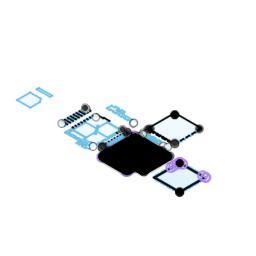
pccases (Autodesk Fusion 360 design; units mm, degrees)
Autodesk Fusion 360 part; units mm, degrees
note: some values were not read from the file. Chosen so that the rebuilt part matches the saved one: which pieces of a blend or face edit are solid.
(part 1 of 5)
sketch "Skizze1" plane through (0, 0, 0) normal (0, 0, 1) x (1, 0, 0)
  line L0 (240, 0) -> (240, 8)
  line L1 (240, 8) -> (10, 8)
  line L2 (10, 8) -> (10, 0)
  line L3 (10.0001, -328) -> (10.0001, -331)
  line L4 (0.0001, -331) -> (0.0001, -328)
  line L5 (250, -328) -> (250, -331)
  line L6 (240, -331) -> (240, -328)
  circle A0 centre (7.5, -7.5) radius 1.5
  circle A1 centre (7.5, -242.5) radius 1.5
  circle A2 centre (242.5, -242.5) radius 1.5
  line L7 (0, 0) -> (10, 0)
  line L8 (0, 0) -> (10, 0)
  line L9 (240, 0) -> (250, 0)
  line L10 (240, -328) -> (10.0001, -328)
  line L11 (10.5, -10.5) -> (239.5, -10.5)
  line L12 (239.5, -10.5) -> (239.5, -239.5)
  line L13 (239.5, -239.5) -> (10.5, -239.5)
  line L14 (10.5, -239.5) -> (10.5, -10.5)
  line L15 (0, -250) -> (-8, -250)
  line L16 (250, -258) -> (250, -250)
  circle A3 centre (-15.5, -7.5) radius 1.5
  circle A4 centre (7.5, -265.5) radius 1.5
  circle A5 centre (242.5, -265.5) radius 1.5
  circle A6 centre (7.5, -320.5) radius 1.5
  circle A7 centre (242.5, -320.5) radius 1.5
  circle A8 centre (-15.5, -242.5) radius 1.5
  circle A9 centre (-70.5, -242.5) radius 1.5
  line L17 (-15, -250) -> (-15, -258)
  line L18 (-15, -258) -> (-22, -258)
  line L19 (-22, -258) -> (-22, -250)
  line L20 (0.0075, -258) -> (-7.9925, -258)
  line L21 (-7.9925, -258) -> (-7.9925, -265)
  line L22 (-7.9925, -265) -> (0, -265)
  line L23 (250, -258) -> (258, -258)
  line L24 (258, -268) -> (250, -268)
  line L25 (250, -250) -> (250, -258)
  line L26 (-15, -250) -> (-8, -250)
  line L27 (-8, -272) -> (-8, -279)
  line L28 (-8, -279) -> (0, -279)
  line L29 (0, -272) -> (-8, -272)
  line L30 (-8, -286) -> (-8, -293)
  line L31 (-8, -293) -> (0, -293)
  line L32 (0, -286) -> (-8, -286)
  line L33 (-8, -300) -> (-8, -307)
  line L34 (-8, -307) -> (0, -307)
  line L35 (0, -300) -> (-8, -300)
  line L36 (-8, -314) -> (-8, -321)
  line L37 (-8, -321) -> (0.0001, -321)
  line L38 (0, -314) -> (-8, -314)
  line L39 (-29, -258) -> (-36, -258)
  line L40 (-36, -258) -> (-36, -250)
  line L41 (-29, -250) -> (-29, -258)
  line L42 (-43, -258) -> (-50, -258)
  line L43 (-50, -258) -> (-50, -250)
  line L44 (-43, -250) -> (-43, -258)
  line L45 (-57, -258) -> (-64, -258)
  line L46 (-64, -258) -> (-64, -250)
  line L47 (-57, -250) -> (-57, -258)
  line L48 (-71, -258) -> (-78, -258)
  line L49 (-78, -258) -> (-78, -250)
  line L50 (-71, -250) -> (-71, -258)
  line L51 (0, -272) -> (0, -265)
  line L52 (0, -286) -> (0, -279)
  line L53 (0, -314) -> (0, -307)
  line L54 (0, -300) -> (0, -293)
  line L55 (250, -318) -> (250, -328)
  line L56 (250, -250) -> (250, -258)
  line L57 (0, 0) -> (-8, 0)
  line L58 (-8, -250) -> (0, -250)
  line L59 (-71, -250) -> (-64, -250)
  line L60 (-57, -250) -> (-50, -250)
  line L61 (-43, -250) -> (-36, -250)
  line L62 (-29, -250) -> (-22, -250)
  line L63 (0, 0) -> (-8, 0)
  line L64 (-78, 8) -> (-8, 8)
  line L65 (250, -250) -> (250, -258)
  line L66 (-18.5, -10.5) -> (-67.5, -10.5)
  line L67 (-67.5, -10.5) -> (-67.5, -239.5)
  line L68 (-67.5, -239.5) -> (-18.5, -239.5)
  line L69 (-18.5, -239.5) -> (-18.5, -10.5)
  circle A10 centre (-70.5, -7.5) radius 1.5
  line L70 (-113.0202, -27.7778) -> (-121, -27.7778)
  line L71 (-113.0173, -55.5556) -> (-121, -55.5556)
  line L72 (-113.0145, -83.3367) -> (-121, -83.3367)
  line L73 (-113.0116, -111.1141) -> (-121, -111.1141)
  line L74 (-113.0087, -138.888) -> (-121, -138.888)
  line L75 (-113.0058, -166.6654) -> (-121, -166.6654)
  line L76 (-113.0029, -194.4429) -> (-121, -194.4429)
  line L77 (-113, -222.2215) -> (-121, -222.2224)
  line L78 (-370.8329, -27.7778) -> (-378.9302, -27.7778)
  line L79 (-370.8329, -55.5556) -> (-378.9302, -55.5556)
  line L80 (-370.8329, -83.3333) -> (-378.9302, -83.3333)
  line L81 (-370.8329, -138.8889) -> (-378.9302, -138.8889)
  line L82 (-370.8329, -166.6667) -> (-378.9302, -166.6667)
  line L83 (-370.8329, -194.4444) -> (-378.9302, -194.4444)
  line L84 (-370.8329, -222.2222) -> (-378.9302, -222.2222)
  line L85 (0, -250) -> (27.7778, -250)
  line L86 (55.5556, -250) -> (83.3333, -250)
  line L87 (111.1111, -250) -> (138.8889, -250)
  line L88 (166.6667, -250) -> (194.4444, -250)
  line L89 (222.2222, -250) -> (250, -250)
  line L90 (-121, -255.9081) -> (-121, -222.2224)
  line L91 (-121, -255.9081) -> (-121, -222.2224)
  line L92 (-121, -194.4429) -> (-121, -166.6654)
  line L93 (-121, -194.4429) -> (-121, -166.6654)
  line L94 (-121, -138.888) -> (-121, -111.1141)
  line L95 (-121, -83.3367) -> (-121, -55.5556)
  line L96 (-121, -138.888) -> (-121, -111.1141)
  line L97 (-121, -83.3367) -> (-121, -55.5556)
  line L98 (-121, -27.7778) -> (-121, 0)
  line L99 (-370.8329, 0) -> (-370.8329, -27.7778)
  line L100 (-370.8329, -55.5556) -> (-370.8329, -83.3333)
  line L101 (-370.8329, -111.1111) -> (-370.8329, -138.8889)
  line L102 (-370.8329, -166.6667) -> (-370.8329, -194.4444)
  line L103 (-370.8329, -222.2222) -> (-370.8329, -263.9081)
  line L104 (10.5, -268.5) -> (239.5, -268.5)
  line L105 (239.5, -268.5) -> (239.5, -317.5)
  line L106 (239.5, -317.5) -> (10.5, -317.5)
  line L107 (10.5, -317.5) -> (10.5, -268.5)
  line L108 (0.0001, -321) -> (0.0001, -328)
  line L109 (0, -27.7778) -> (-8, -27.7778)
  line L110 (0, -55.5556) -> (-8, -55.5556)
  line L111 (0, -83.3333) -> (-8, -83.3333)
  line L112 (0, -111.1111) -> (-8, -111.1111)
  line L113 (0, -138.8889) -> (-8, -138.8889)
  line L114 (0, -166.6667) -> (-8, -166.6667)
  line L115 (0, -194.4444) -> (-8, -194.4444)
  line L116 (0, -222.2222) -> (-8, -222.2222)
  line L117 (0, -250) -> (-8, -250)
  line L118 (-8, -27.7778) -> (-8, -55.5556)
  line L119 (-8, -83.3333) -> (-8, -111.1111)
  line L120 (-8, -138.8889) -> (-8, -166.6667)
  line L121 (-8, -194.4444) -> (-8, -222.2222)
  line L122 (0, -222.2222) -> (0.0075, -258)
  line L123 (0, -111.1111) -> (0, -138.8889)
  line L124 (0, -166.6667) -> (0, -194.4444)
  line L125 (0, 0) -> (0, -27.7778)
  line L126 (0, -55.5556) -> (0, -83.3333)
  line L127 (-78, -27.7778) -> (-86, -27.7778)
  line L128 (-78, -55.5556) -> (-86, -55.5556)
  line L129 (-78, -83.3333) -> (-86, -83.3333)
  line L130 (-78, -111.1111) -> (-86, -111.1111)
  line L131 (-78, -138.8889) -> (-86, -138.8889)
  line L132 (-78, -166.6667) -> (-86, -166.6667)
  line L133 (-78, -194.4444) -> (-86, -194.4444)
  line L134 (-78, -222.2222) -> (-86, -222.2222)
  line L135 (-355.7398, -242.9081) -> (-228.7398, -242.9081)
  line L136 (-228.7398, -242.9081) -> (-228.7398, -263.9081)
  line L137 (-355.7398, -263.9081) -> (-355.7398, -242.9081)
  line L138 (-253.6584, -13) -> (-253.6584, 8)
  line L139 (-126.6584, -0.0224) -> (-126.6584, -13)
  line L140 (-126.6584, -13) -> (-253.6584, -13)
  line L141 (-355.7398, -116.9081) -> (-253.7398, -116.9081)
  line L142 (-228.7398, -152.9081) -> (-228.7398, -242.9081)
  line L143 (-228.7398, -242.9081) -> (-355.7398, -242.9081)
  line L144 (-355.7398, -242.9081) -> (-355.7398, -116.9081)
  line L145 (-253.7398, -116.9081) -> (-228.7398, -152.9081)
  line L146 (-739.7286, -77.336) -> (-866.7286, -77.336)
  line L147 (-739.7286, -56.336) -> (-739.7286, -77.336)
  line L148 (-866.7286, -56.336) -> (-739.7286, -56.336)
  line L149 (-866.7286, -77.336) -> (-866.7286, -56.336)
  line L150 (-253.6584, -13) -> (-126.6584, -13)
  line L151 (-126.6584, -139) -> (-228.6584, -139)
  line L152 (-126.6584, -13) -> (-126.6584, -139)
  line L153 (-228.6584, -139) -> (-253.6584, -103)
  line L154 (-253.6584, -103) -> (-253.6584, -13)
  line L155 (-769.2291, -135.4616) -> (-744.2291, -171.4616)
  line L156 (-744.2291, -261.4616) -> (-871.2291, -261.4616)
  line L157 (-871.2291, -135.4616) -> (-769.2291, -135.4616)
  line L158 (-871.2291, -261.4616) -> (-871.2291, -135.4616)
  line L159 (-744.2291, -171.4616) -> (-744.2291, -261.4616)
  line L160 (-272.1218, -90.438) -> (-217.7916, -168.6735)
  line L161 (-217.7916, -168.6735) -> (-211.2206, -164.1103)
  line L162 (-211.2206, -164.1103) -> (-265.5508, -85.8749)
  line L163 (-265.5508, -85.8749) -> (-272.1218, -90.438)
  line L164 (-166.6477, -255.9081) -> (-121, -255.9081)
  line L165 (-306.8112, 0) -> (-370.8329, 0)
  line L166 (-355.7398, -263.9081) -> (-370.8329, -263.9081)
  line L167 (-306.8112, 8) -> (-306.8112, 0)
  line L168 (-166.6477, -255.9081) -> (-166.6477, -263.9081)
  line L169 (-43, 3) -> (-43, 6)
  line L170 (317.5, -239.5) -> (268.5, -239.5)
  line L171 (258, -250) -> (250, -250)
  circle A11 centre (320.5, -242.5) radius 1.5
  line L172 (250, -240) -> (258, -240)
  circle A12 centre (265.5, -242.5) radius 1.5
  circle A13 centre (265.5, -7.5) radius 1.5
  line L173 (250, 0) -> (258, -0.0533)
  line L174 (250, -10.0533) -> (258, -10.0533)
  line L175 (268.5, -10.5) -> (317.5, -10.5)
  line L176 (250, 8) -> (250, 0)
  circle A14 centre (320.5, -7.5) radius 1.5
  line L177 (328, 8) -> (258, 8)
  line L178 (250, -250) -> (258, -250)
  line L179 (250, -250) -> (258, -250)
  line L180 (268.5, -239.5) -> (268.5, -10.5)
  line L181 (317.5, -10.5) -> (317.5, -239.5)
  line L182 (55.5556, -258) -> (27.7778, -258)
  line L183 (111.1111, -258) -> (83.3333, -258)
  line L184 (166.6667, -258) -> (138.8889, -258)
  line L185 (222.2222, -258) -> (194.4444, -258)
  line L186 (27.7778, -258) -> (27.7778, -250)
  line L187 (55.5556, -258) -> (55.5556, -250)
  line L188 (83.3333, -258) -> (83.3333, -250)
  line L189 (111.1111, -258) -> (111.1111, -250)
  line L190 (166.6667, -258) -> (166.6667, -250)
  line L191 (138.8889, -258) -> (138.8889, -250)
  line L192 (194.4444, -258) -> (194.4444, -250)
  line L193 (222.2222, -258) -> (222.2222, -250)
  line L194 (-121, 8) -> (-121, 0)
  line L195 (-126.6584, -0.0224) -> (-126.6584, 8)
  line L196 (-378.9302, -55.5556) -> (-378.9302, -27.7778)
  line L197 (-378.9302, -111.1111) -> (-378.9302, -83.3333)
  line L198 (-378.9302, -222.2222) -> (-378.9302, -194.4444)
  line L199 (-378.9302, -166.6667) -> (-378.9302, -138.8889)
  line L200 (258, -240) -> (258, -10.0533)
  line L201 (250, 0) -> (250, -10.0533)
  line L202 (250, -240) -> (250, -250)
  line L203 (448.7457, -6) -> (655.1901, -6)
  line L204 (670.9679, -21.7778) -> (670.9679, -228.2222)
  line L205 (655.1901, -244) -> (448.7457, -244)
  line L206 (432.9679, -228.2222) -> (432.9679, -21.7778)
  line L207 (328, 0) -> (336, 0)
  line L208 (336, -250.0403) -> (328, -250.0403)
  line L209 (328, -27.7778) -> (336, -27.7778)
  line L210 (328, -55.5556) -> (336, -55.5556)
  line L211 (328, -83.3333) -> (336, -83.3333)
  line L212 (328, -111.1111) -> (336, -111.1111)
  line L213 (328, -138.8889) -> (336, -138.8889)
  line L214 (328, -166.6667) -> (336, -166.6667)
  line L215 (328, -194.4444) -> (336, -194.4444)
  line L216 (328, -222.2222) -> (336, -222.2222)
  line L217 (328, -250) -> (336, -250)
  circle A15 centre (-350.3021, -25.5485) radius 6
  line L218 (-113.0202, -27.7778) -> (-113.0173, -55.5556)
  line L219 (-113.0145, -83.3367) -> (-113.0116, -111.1141)
  line L220 (-113.0087, -138.888) -> (-113.0058, -166.6654)
  line L221 (-113.0029, -194.4429) -> (-113, -222.2215)
  line L222 (-228.7398, -309.2127) -> (-228.7398, -322.2127)
  line L223 (-228.7398, -309.2127) -> (-166.6477, -309.2127)
  line L224 (-166.6477, -301.2127) -> (-166.6477, -309.2127)
  line L225 (-202.1286, -333.2127) -> (-202.1286, -322.2127)
  line L226 (-177.4668, -333.2127) -> (-177.4668, -322.2127)
  line L227 (-146.2286, -333.2127) -> (-146.2286, -322.2127)
  line L228 (-228.7398, -309.2127) -> (-166.6477, -309.2127)
  line L229 (-121, -322.2127) -> (-121, -282.214)
  line L230 (-166.6477, -301.2127) -> (-228.7398, -301.214)
  line L231 (-306.8112, 8) -> (-253.6584, 8)
  line L232 (-126.6584, 8) -> (-121, 8)
  line L233 (-228.7398, -263.9081) -> (-166.6477, -263.9081)
  line L234 (-370.8329, -263.9081) -> (-355.7398, -263.9081)
  line L235 (-257.7401, 156.9081) -> (-257.7401, 145.9081)
  line L236 (-306.8112, 135.9081) -> (-253.6584, 135.9081)
  line L237 (-370.8022, 145.9081) -> (-370.8022, 108.9086)
  line L238 (-312.3976, 156.9081) -> (-312.3976, 145.9081)
  line L239 (-306.8112, 135.9081) -> (-306.8112, 127.9081)
  line L240 (-340.8694, 156.9081) -> (-340.8694, 145.9081)
  line L241 (-285.3527, 156.9081) -> (-285.3527, 145.9081)
  line L242 (-253.6584, 145.9081) -> (-253.6584, 135.9081)
  line L243 (-306.8112, 127.9081) -> (-120.8022, 127.9081)
  line L244 (-370.8329, -290.214) -> (-370.8329, -301.214)
  line L245 (-370.8329, -301.214) -> (-228.7398, -301.214)
  line L246 (-370.8329, -282.214) -> (-370.8329, -290.214)
  line L247 (-343.0551, -282.214) -> (-343.0551, -290.214)
  line L248 (-315.2773, -282.214) -> (-315.2773, -290.214)
  line L249 (-287.4996, -282.214) -> (-287.4996, -290.214)
  line L250 (-259.7218, -282.214) -> (-259.7218, -290.214)
  line L251 (-231.944, -282.214) -> (-231.944, -290.214)
  line L252 (-204.1662, -282.214) -> (-204.1662, -290.214)
  line L253 (-176.3884, -282.214) -> (-176.3884, -290.214)
  line L254 (-148.6107, -282.214) -> (-148.6107, -290.214)
  line L255 (-120.8022, 116.9081) -> (-120.8022, 100.9086)
  line L256 (-370.8022, 100.9086) -> (-370.8022, 108.9086)
  line L257 (-120.8022, 127.9081) -> (-120.8022, 116.9081)
  line L258 (-343.0244, 100.9086) -> (-343.0244, 108.9086)
  line L259 (-315.2466, 100.9086) -> (-315.2466, 108.9086)
  line L260 (-287.4688, 100.9086) -> (-287.4688, 108.9086)
  line L261 (-259.6911, 100.9086) -> (-259.6911, 108.9086)
  line L262 (-231.9133, 100.9086) -> (-231.9133, 108.9086)
  line L263 (-204.1355, 100.9086) -> (-204.1355, 108.9086)
  line L264 (-176.3577, 100.9086) -> (-176.3577, 108.9086)
  line L265 (-148.5799, 100.9086) -> (-148.5799, 108.9086)
  line L266 (-120.8022, 100.9086) -> (-120.8022, 108.9086)
  line L267 (-343.0244, 108.9086) -> (-315.2466, 108.9086)
  line L268 (-176.3577, 108.9086) -> (-148.5799, 108.9086)
  line L269 (-287.4688, 108.9086) -> (-259.6911, 108.9086)
  line L270 (-231.9133, 108.9086) -> (-204.1355, 108.9086)
  line L271 (-343.0244, 100.9086) -> (-370.8022, 100.9086)
  line L272 (-287.4688, 100.9086) -> (-315.2466, 100.9086)
  line L273 (-231.9133, 100.9086) -> (-259.6911, 100.9086)
  line L274 (-120.8022, 100.9086) -> (-148.5799, 100.9086)
  line L275 (-176.3577, 100.9086) -> (-204.1355, 100.9086)
  line L276 (418.9679, -222.2222) -> (426.9679, -222.2222)
  line L277 (684.9679, -222.2222) -> (676.9679, -222.2222)
  line L278 (418.9679, -194.4444) -> (426.9679, -194.4444)
  line L279 (684.9679, -194.4444) -> (676.9679, -194.4444)
  line L280 (418.9679, -166.6667) -> (426.9679, -166.6667)
  line L281 (684.9679, -166.6667) -> (676.9679, -166.6667)
  line L282 (418.9679, -138.8889) -> (426.9679, -138.8889)
  line L283 (684.9679, -138.8889) -> (676.9679, -138.8889)
  line L284 (418.9679, -111.1111) -> (426.9679, -111.1111)
  line L285 (684.9679, -111.1111) -> (676.9679, -111.1111)
  line L286 (418.9679, -83.3333) -> (426.9679, -83.3333)
  line L287 (684.9679, -83.3333) -> (676.9679, -83.3333)
  line L288 (418.9679, -55.5556) -> (426.9679, -55.5556)
  line L289 (684.9679, -55.5556) -> (676.9679, -55.5556)
  line L290 (418.9679, -27.7778) -> (426.9679, -27.7778)
  line L291 (684.9679, -27.7778) -> (676.9679, -27.7778)
  line L292 (454.7457, -258) -> (454.7457, -250)
  line L293 (454.7457, 8) -> (454.7457, 0)
  line L294 (482.5234, -258) -> (482.5234, -250)
  line L295 (482.5234, 8) -> (482.5234, 0)
  line L296 (510.3012, -258) -> (510.3012, -250)
  line L297 (510.3012, 8) -> (510.3012, 0)
  line L298 (538.079, -258) -> (538.079, -250)
  line L299 (538.079, 8) -> (538.079, 0)
  line L300 (565.8568, -258) -> (565.8568, -250)
  line L301 (565.8568, 8) -> (565.8568, 0)
  line L302 (593.6346, -258) -> (593.6346, -250)
  line L303 (593.6346, 8) -> (593.6346, 0)
  line L304 (621.4123, -258) -> (621.4123, -250)
  line L305 (621.4123, 8) -> (621.4123, 0)
  line L306 (649.1901, -258) -> (649.1901, -250)
  line L307 (649.1901, 8) -> (649.1901, 0)
  line L308 (482.5234, -258) -> (454.7457, -258)
  line L309 (538.079, -258) -> (510.3012, -258)
  line L310 (649.1901, -258) -> (621.4123, -258)
  line L311 (593.6346, -258) -> (565.8568, -258)
  line L312 (684.9679, -194.4444) -> (684.9679, -222.2222)
  line L313 (684.9679, -138.8889) -> (684.9679, -166.6667)
  line L314 (684.9679, -27.7778) -> (684.9679, -55.5556)
  line L315 (684.9679, -83.3333) -> (684.9679, -111.1111)
  line L316 (649.1901, 8) -> (621.4123, 8)
  line L317 (593.6346, 8) -> (565.8568, 8)
  line L318 (538.079, 8) -> (510.3012, 8)
  line L319 (482.5234, 8) -> (454.7457, 8)
  line L320 (418.9679, -27.7778) -> (418.9679, -55.5556)
  line L321 (418.9679, -83.3333) -> (418.9679, -111.1111)
  line L322 (418.9679, -138.8889) -> (418.9679, -166.6667)
  line L323 (418.9679, -194.4444) -> (418.9679, -222.2222)
  line L324 (426.9679, -83.3333) -> (426.9679, -55.5556)
  line L325 (426.9679, -27.7778) -> (426.9679, 0)
  line L326 (426.9679, -83.3333) -> (426.9679, -55.5556)
  line L327 (426.9679, -27.7778) -> (426.9679, 0)
  line L328 (426.9679, -138.8889) -> (426.9679, -111.1111)
  line L329 (426.9679, -138.8889) -> (426.9679, -111.1111)
  line L330 (426.9679, -250) -> (426.9679, -222.2222)
  line L331 (426.9679, -194.4444) -> (426.9679, -166.6667)
  line L332 (426.9679, -250) -> (426.9679, -222.2222)
  line L333 (426.9679, -194.4444) -> (426.9679, -166.6667)
  line L334 (454.7457, -250) -> (426.9679, -250)
  line L335 (426.9679, -250) -> (454.7457, -250)
  line L336 (482.5234, -250) -> (510.3012, -250)
  line L337 (510.3012, -250) -> (482.5234, -250)
  line L338 (565.8568, -250) -> (538.079, -250)
  line L339 (538.079, -250) -> (565.8568, -250)
  line L340 (676.9679, -250) -> (649.1901, -250)
  line L341 (621.4123, -250) -> (593.6346, -250)
  line L342 (593.6346, -250) -> (621.4123, -250)
  line L343 (649.1901, -250) -> (676.9679, -250)
  line L344 (676.9679, -250) -> (676.9679, -222.2222)
  line L345 (676.9679, -222.2222) -> (676.9679, -250)
  line L346 (676.9679, -27.7778) -> (676.9679, 0)
  line L347 (676.9679, 0) -> (676.9679, -27.7778)
  line L348 (676.9679, -55.5556) -> (676.9679, -83.3333)
  line L349 (676.9679, -83.3333) -> (676.9679, -55.5556)
  line L350 (676.9679, -194.4444) -> (676.9679, -166.6667)
  line L351 (676.9679, -138.8889) -> (676.9679, -111.1111)
  line L352 (676.9679, -111.1111) -> (676.9679, -138.8889)
  line L353 (676.9679, -166.6667) -> (676.9679, -194.4444)
  line L354 (649.1901, 0) -> (676.9679, 0)
  line L355 (593.6346, 0) -> (621.4123, 0)
  line L356 (482.5234, 0) -> (510.3012, 0)
  line L357 (538.079, 0) -> (565.8568, 0)
  line L358 (426.9679, 0) -> (454.7457, 0)
  line L359 (-343.0551, -290.214) -> (-315.2773, -290.214)
  line L360 (-315.2773, -290.214) -> (-343.0551, -290.214)
  line L361 (-148.6107, -290.214) -> (-176.3884, -290.214)
  line L362 (-287.4996, -290.214) -> (-259.7218, -290.214)
  line L363 (-204.1662, -290.214) -> (-231.944, -290.214)
  line L364 (-259.7218, -290.214) -> (-287.4996, -290.214)
  line L365 (-231.944, -290.214) -> (-204.1662, -290.214)
  line L366 (-176.3884, -290.214) -> (-148.6107, -290.214)
  line L367 (-343.0551, -282.214) -> (-370.8329, -282.214)
  line L368 (-121, -282.214) -> (-148.6107, -282.214)
  line L369 (-176.3884, -282.214) -> (-204.1662, -282.214)
  line L370 (-231.944, -282.214) -> (-259.7218, -282.214)
  line L371 (-287.4996, -282.214) -> (-315.2773, -282.214)
  line L372 (328, -55.5556) -> (328, -27.7778)
  line L373 (328, -27.7778) -> (328, -55.5556)
  line L374 (328, -83.3333) -> (328, -111.1111)
  line L375 (328, -111.1111) -> (328, -83.3333)
  line L376 (328, -166.6667) -> (328, -138.8889)
  line L377 (328, -138.8889) -> (328, -166.6667)
  line L378 (328, -194.4444) -> (328, -222.2222)
  line L379 (328, -250.0403) -> (328, -250)
  line L380 (328, -222.2222) -> (328, -194.4444)
  line L381 (336, -222.2222) -> (336, -250.0403)
  line L382 (336, -250.0403) -> (336, -222.2222)
  line L383 (336, -194.4444) -> (336, -166.6667)
  line L384 (336, -166.6667) -> (336, -194.4444)
  line L385 (336, -111.1111) -> (336, -138.8889)
  line L386 (336, 0) -> (336, -27.7778)
  line L387 (336, -55.5556) -> (336, -83.3333)
  line L388 (336, -83.3333) -> (336, -55.5556)
  line L389 (336, -27.7778) -> (336, 0)
  line L390 (-455.7798, -222.2222) -> (-455.7798, -194.4444)
  line L391 (-468.7798, -194.4444) -> (-479.7798, -194.4444)
  line L392 (-447.7798, -27.7778) -> (-455.7798, -27.7778)
  line L393 (-468.7798, -27.7778) -> (-479.7798, -27.7778)
  line L394 (-447.7798, -55.5556) -> (-455.7798, -55.5556)
  line L395 (-468.7798, -55.5556) -> (-479.7798, -55.5556)
  line L396 (-447.7798, -83.3333) -> (-455.7798, -83.3333)
  line L397 (-455.7798, -55.5556) -> (-455.7798, -27.7778)
  line L398 (-455.7798, -111.1111) -> (-455.7798, -83.3333)
  line L399 (-468.7798, -83.3333) -> (-479.7798, -83.3333)
  line L400 (-468.7798, 0) -> (-436.3953, 0)
  line L401 (-447.7798, -194.4444) -> (-455.7798, -194.4444)
  line L402 (-455.7798, -166.6667) -> (-455.7798, -138.8889)
  line L403 (-447.7798, -166.6667) -> (-455.7798, -166.6667)
  line L404 (-468.7798, -138.8889) -> (-479.7798, -138.8889)
  line L405 (-447.7798, -111.1111) -> (-455.7798, -111.1111)
  line L406 (-468.7798, -111.1111) -> (-479.7798, -111.1111)
  line L407 (-468.7798, -166.6667) -> (-479.7798, -166.6667)
  line L408 (-468.7798, -222.2222) -> (-479.7798, -222.2222)
  line L409 (-447.7798, -138.8889) -> (-455.7798, -138.8889)
  line L410 (-455.7798, -222.2222) -> (-447.7798, -222.2222)
  line L411 (-436.3953, 0) -> (-468.7798, 0)
  line L412 (-436.3953, 0) -> (-428.3953, 0)
  line L413 (-436.3953, -27.7778) -> (-428.3953, -27.7778)
  line L414 (-436.3953, -55.5556) -> (-428.3953, -55.5556)
  line L415 (-436.3953, -83.3333) -> (-428.3953, -83.3333)
  line L416 (-436.3953, -111.1111) -> (-428.3953, -111.1111)
  line L417 (-436.3953, -138.8889) -> (-428.3953, -138.8889)
  line L418 (-436.3953, -166.6667) -> (-428.3953, -166.6667)
  line L419 (-436.3953, -194.4444) -> (-428.3953, -194.4444)
  line L420 (-436.3953, -222.2222) -> (-428.3953, -222.2222)
  line L421 (-447.7798, -27.7778) -> (-447.7798, -55.5556)
  line L422 (-447.7798, -83.3333) -> (-447.7798, -111.1111)
  line L423 (-447.7798, -138.8889) -> (-447.7798, -166.6667)
  line L424 (-447.7798, -194.4444) -> (-447.7798, -222.2222)
  line L425 (-436.3953, -55.5556) -> (-436.3953, -27.7778)
  line L426 (-436.3953, -55.5556) -> (-436.3953, -27.7778)
  line L427 (-436.3953, -111.1111) -> (-436.3953, -83.3333)
  line L428 (-436.3953, -111.1111) -> (-436.3953, -83.3333)
  line L429 (-436.3953, -166.6667) -> (-436.3953, -138.8889)
  line L430 (-436.3953, -166.6667) -> (-436.3953, -138.8889)
  line L431 (-428.3953, 0) -> (-428.3953, -27.7778)
  line L432 (-428.3953, -55.5556) -> (-428.3953, -83.3333)
  line L433 (-428.3953, -111.1111) -> (-428.3953, -138.8889)
  line L434 (-428.3953, -166.6667) -> (-428.3953, -194.4444)
  line L435 (-428.3953, -222.2222) -> (-428.3953, -250)
  line L436 (-436.3953, -222.2222) -> (-436.3953, -194.4444)
  line L437 (-436.3953, -222.2222) -> (-436.3953, -194.4444)
  line L438 (-378.9302, -111.1111) -> (-370.8329, -111.1111)
  line L439 (482.5234, 0) -> (510.3012, 0)
  line L440 (538.079, 0) -> (565.8568, 0)
  line L441 (593.6346, 0) -> (621.4123, 0)
  line L442 (649.1901, 0) -> (676.9679, 0)
  line L443 (-428.3953, -250) -> (-468.7798, -250)
  line L444 (320.2222, 2.5) -> (320.2222, 5.5)
  line L445 (312.4444, 2.5) -> (312.4444, 5.5)
  line L446 (304.6666, 2.5) -> (304.6666, 5.5)
  line L447 (296.8889, 2.5) -> (296.8889, 5.5)
  line L448 (289.1111, 2.5) -> (289.1111, 5.5)
  line L449 (273.5555, 2.5) -> (273.5555, 5.5)
  line L450 (265.7778, 2.5) -> (265.7778, 5.5)
  line L451 (281.3333, 2.5) -> (281.3333, 5.5)
  line L452 (265.7778, 5.5) -> (258, 5.5)
  line L453 (258, 2.5) -> (265.7778, 2.5)
  line L454 (281.3333, 5.5) -> (273.5555, 5.5)
  line L455 (273.5555, 2.5) -> (281.3333, 2.5)
  line L456 (296.8889, 5.5) -> (289.1111, 5.5)
  line L457 (289.1111, 2.5) -> (296.8889, 2.5)
  line L458 (328, 5.5) -> (320.2222, 5.5)
  line L459 (312.4444, 5.5) -> (304.6666, 5.5)
  line L460 (304.6666, 2.5) -> (312.4444, 2.5)
  line L461 (320.2222, 2.5) -> (328, 2.5)
  line L462 (250, 0) -> (258, 0)
  line L463 (328, 0) -> (328, 2.5)
  line L464 (328, 5.5) -> (328, 8)
  line L465 (258, -0.0533) -> (258, 2.5)
  line L466 (258, 5.5) -> (258, 8)
  line L467 (328, -0.0533) -> (328, 2.5)
  line L468 (328, 5.5) -> (328, 8)
  line L469 (268, -250) -> (268, -258)
  line L470 (268, -258) -> (258, -258)
  line L471 (258, -258) -> (258, -250)
  line L472 (318, -250) -> (318, -258)
  line L473 (318, -258) -> (328, -258)
  line L474 (328, -258) -> (328, -250)
  line L475 (268, -250) -> (318, -250)
  line L476 (250, -318) -> (258, -318)
  line L477 (250, -258) -> (250, -268)
  line L478 (250, -318) -> (250, -321)
  line L479 (-8, 0) -> (-8, 3)
  line L480 (-8, 6) -> (-8, 8)
  line L481 (-78, -250) -> (-86, -250)
  line L482 (-78, 0) -> (-86, 0)
  line L483 (-78, -194.4444) -> (-78, -222.2222)
  line L484 (-86, -222.2222) -> (-86, -250)
  line L485 (-86, -166.6667) -> (-86, -194.4444)
  line L486 (-78, -138.8889) -> (-78, -166.6667)
  line L487 (-78, -27.7778) -> (-78, -55.5556)
  line L488 (-78, -83.3333) -> (-78, -111.1111)
  line L489 (-86, -111.1111) -> (-86, -138.8889)
  line L490 (-86, 0) -> (-86, -27.7778)
  line L491 (-86, -55.5556) -> (-86, -83.3333)
  line L492 (-479.7798, -27.7778) -> (-479.7798, -55.5556)
  line L493 (-479.7798, -83.3333) -> (-479.7798, -111.1111)
  line L494 (-479.7798, -138.8889) -> (-479.7798, -166.6667)
  line L495 (-479.7798, -194.4444) -> (-479.7798, -222.2222)
  line L496 (-468.7798, -138.8889) -> (-468.7798, -111.1111)
  line L497 (-468.7798, -250) -> (-468.7798, -222.2222)
  line L498 (-468.7798, -194.4444) -> (-468.7798, -166.6667)
  line L499 (-468.7798, -83.3333) -> (-468.7798, -55.5556)
  line L500 (-468.7798, -27.7778) -> (-468.7798, 0)
  line L501 (250, -331) -> (250, -339)
  line L502 (0.0001, -339) -> (0.0001, -331)
  line L503 (27.7779, -339) -> (27.7779, -331)
  line L504 (222.2223, -339) -> (222.2223, -331)
  line L505 (250.0001, -339) -> (250.0001, -331)
  line L506 (250, -331) -> (250.0001, -331)
  line L507 (240.0016, -331) -> (240, -331)
  line L508 (250, -339) -> (222.2223, -339)
  line L509 (27.7779, -339) -> (0.0001, -339)
  line L510 (10.0001, -331) -> (27.7779, -331)
  line L511 (222.2223, -331) -> (240.0016, -331)
  line L512 (-340.8694, 156.9081) -> (-312.3976, 156.9081)
  line L513 (-285.3527, 156.9081) -> (-257.7401, 156.9081)
  line L514 (-253.6584, 145.9081) -> (-257.7401, 145.9081)
  line L515 (-285.3527, 145.9081) -> (-312.3976, 145.9081)
  line L516 (-340.8694, 145.9081) -> (-370.8022, 145.9081)
  line L517 (-228.7398, -322.2127) -> (-228.7398, -333.2127)
  line L518 (-146.2286, -333.2127) -> (-177.4668, -333.2127)
  line L519 (-202.1286, -333.2127) -> (-228.7398, -333.2127)
  line L520 (-121, -322.2127) -> (-146.2286, -322.2127)
  line L521 (-177.4668, -322.2127) -> (-202.1286, -322.2127)
  circle A16 centre (-461.2792, -7.5001) radius 1.5
  circle A17 centre (-461.2799, -242.5026) radius 1.5
  line L522 (-8, 6) -> (-8, 3)
  line L523 (-43, 3) -> (-78, 3)
  line L524 (-43, 6) -> (-78, 6)
  line L525 (-78, 0) -> (-78, 3)
  line L526 (-78, 6) -> (-78, 8)
  line L527 (432.9679, -228.2222) -> (448.7457, -244)
  line L528 (655.1901, -6) -> (670.9679, -21.7778)
  line L529 (448.7457, -6) -> (432.9679, -21.7778)
  line L530 (670.9679, -228.2222) -> (655.1901, -244)
  point P0 (-121, 0)
  point P1 (328, -250)
  point P2 (328, -250)
  point P3 (250, 0)
  point P4 (250, 0)
  point P5 (328, -250)
  point P6 (328, -250)
  point P7 (250, 0)
  point P8 (328, 0)
  point P9 (-479.7798, 0)
  point P10 (-479.7798, 0)
  point P11 (250, -321)
  dimension "d12" = 250
  dimension "d13" = 250
  dimension "d19" = 78
  dimension "d20" = 78
  dimension "longnotch_l" = 230
  dimension "d23" = 8
  dimension "d52" = 10
  dimension "d60" = 3
  dimension "d76" = 3
  dimension "d77" = 7.5
  dimension "d78" = 7.5
  dimension "d84" = 235
  dimension "d113" = 10.5
  dimension "d114" = 10.5
  dimension "d115" = 10.5
  dimension "d116" = 10.5
  dimension "d183" = 8
  dimension "d263" = 235
  dimension "d270" = 15.5
  dimension "d271" = 15.5
  dimension "d272" = 7.5
  dimension "d274" = 7.5
  dimension "sidenub_l" = 7
  dimension "d278" = 8
  dimension "d298" = 8
  dimension "d299" = 8
  dimension "d348" = 7
  dimension "d349" = 7
  dimension "d357" = -14
  dimension "d358" = 0
  dimension "d371" = 78
  dimension "d411" = 10
  dimension "d592" = 10
  dimension "d593" = 10
  dimension "d607" = 10.5
  dimension "d608" = 10.5
  dimension "d677" = 18.5
  dimension "d678" = 10.5
  dimension "d680" = 10.5
  dimension "d681" = 10.5
  dimension "d684" = 10.5
  dimension "d688" = 0
  dimension "d692" = 127
  dimension "d693" = 21
  dimension "d699" = 126
  dimension "d702" = 25
  dimension "d703" = 36
  dimension "d704" = 127
  dimension "d705" = 127
  dimension "d706" = 21
  dimension "d707" = 126
  dimension "d710" = 127
  dimension "d711" = 126
  dimension "d712" = 25
  dimension "d713" = 36
  dimension "d714" = 127
  dimension "d715" = 25
  dimension "d716" = 36
  dimension "d718" = 8
  dimension "d719" = 95.25
  dimension "d742" = 8
  dimension "d743" = 8
  dimension "d816" = 250
  dimension "d817" = 250
  dimension "d820" = 6
  dimension "d821" = 6
  dimension "d826" = 8
  dimension "d833" = 12
  dimension "d840" = 8
  dimension "d841" = 8
  dimension "d843" = 13
  dimension "d848" = 8
  dimension "d854" = 11
  dimension "d856" = 8
  dimension "d859" = 250
  dimension "d860" = 0
  dimension "d862" = 8
  dimension "d865" = 250
  dimension "d866" = 0
  dimension "d867" = 11
  dimension "d868" = 250
  dimension "d884" = 11
  dimension "d885" = 13
  dimension "d887" = 8
  dimension "d890" = 8
  dimension "d893" = 0
  dimension "d896" = 242.9081
  dimension "d921" = 8
  dimension "d922" = 2.5
  dimension "d923" = 3
  dimension "d929" = 10
  dimension "d930" = 8
  dimension "d931" = 10
  dimension "d932" = 8
  dimension "d933" = 10
  dimension "d934" = 8
  dimension "d937" = 8
  dimension "d938" = 35
  dimension "d948" = 8
  dimension "d949" = 8
  dimension "d951" = 8
  dimension "d954" = 250
  dimension "d955" = 0
  dimension "d956" = 10
  dimension "d1024" = 3
  dimension "d1025" = 3
  dimension "d1026" = 3.5404
  dimension "d1027" = 4.256
  dimension "d1028" = 7.2978
  dimension "d1029" = 5.6908
  dimension "d1031" = 3
  constraint horizontal L8
  constraint coincident L7.start L8.start
  constraint horizontal L7
  constraint horizontal L59
  constraint vertical L25
  constraint vertical L0
  constraint horizontal L1
  constraint vertical L2
  constraint vertical L3
  constraint vertical L4
  constraint vertical L5
  constraint horizontal L506
  constraint vertical L6
  constraint collinear L8 L9
  constraint horizontal L11
  constraint vertical L12
  constraint horizontal L13
  constraint vertical L14
  constraint horizontal L15
  constraint vertical L16
  constraint equal A3 A4
  constraint equal A0 A4
  constraint vertical L17
  constraint horizontal L18
  constraint vertical L19
  constraint horizontal L20
  constraint vertical L21
  constraint horizontal L22
  constraint horizontal L23
  constraint horizontal L24
  constraint collinear L26 L59
  constraint coincident L5.start L55.end
  constraint coincident L15.end L26.end
  constraint coincident L16.start L23.start
  constraint coincident L28 L52.end
  constraint coincident L29 L51.start
  constraint coincident L31 L54.end
  constraint coincident L32 L52.start
  constraint coincident L38 L53.start
  constraint coincident L34 L53.end
  constraint coincident L35 L54.start
  constraint vertical L56
  constraint horizontal L57
  constraint horizontal L58
  constraint collinear L59 L60
  constraint collinear L60 L61
  constraint collinear L61 L62
  constraint horizontal L63
  constraint vertical L525
  constraint horizontal L64
  constraint vertical L118
  constraint coincident L15.start L58.end
  constraint horizontal L10
  constraint equal L20 L58
  constraint collinear L20 L23
  constraint coincident L16.end L25.start
  constraint horizontal L85
  constraint vertical L65
  constraint horizontal L66
  constraint vertical L67
  constraint horizontal L68
  constraint vertical L69
  constraint vertical L91
  constraint vertical L90
  constraint coincident P0 L98.end
  constraint collinear L85 L86
  constraint collinear L86 L87
  constraint collinear L87 L88
  constraint collinear L88 L89
  constraint collinear L90 L93
  constraint collinear L91 L92
  constraint collinear L92 L96
  constraint collinear L93 L94
  constraint collinear L94 L95
  constraint collinear L96 L97
  constraint collinear L97 L98
  constraint collinear L99 L100
  constraint collinear L100 L101
  constraint collinear L101 L102
  constraint collinear L102 L103
  constraint horizontal L104
  constraint vertical L105
  constraint horizontal L106
  constraint vertical L107
  constraint equal L3 L4
  constraint equal L4 L6
  constraint equal L5 L6
  constraint collinear L51 L125
  constraint collinear L118 L120
  constraint collinear L118 L119
  constraint collinear L120 L121
  constraint collinear L123 L125
  constraint collinear L123 L124
  constraint collinear L125 L126
  constraint horizontal L135
  constraint vertical L136
  constraint vertical L137
  constraint vertical L139
  constraint horizontal L140
  constraint vertical L138
  constraint equal L137 L138
  constraint horizontal L141
  constraint vertical L142
  constraint horizontal L143
  constraint vertical L144
  constraint coincident L99.start L165.end
  constraint horizontal L148
  constraint vertical L147
  constraint horizontal L146
  constraint vertical L149
  constraint horizontal L157
  constraint vertical L159
  constraint horizontal L156
  constraint vertical L158
  constraint vertical L154
  constraint horizontal L150
  constraint vertical L152
  constraint horizontal L151
  constraint perpendicular L160 L161
  constraint perpendicular L161 L162
  constraint parallel L161 L163
  constraint collinear L153 L162
  constraint collinear L145 L160
  constraint horizontal L164
  constraint vertical L169
  constraint coincident L29.start L51.start
  constraint coincident L28.end L52.end
  constraint coincident L32.start L52.start
  constraint coincident L31.end L54.end
  constraint coincident L35.start L54.start
  constraint coincident L34.end L53.end
  constraint coincident L38.start L53.start
  constraint vertical L180
  constraint vertical L181
  constraint horizontal L179
  constraint vertical L463
  constraint vertical L176
  constraint horizontal L462
  constraint horizontal L177
  constraint horizontal L175
  constraint horizontal L170
  constraint horizontal L172
  constraint coincident P7 P4
  constraint coincident P6 P5
  constraint coincident L171.start L178.end
  constraint horizontal L174
  constraint symmetric L186.end L85 L85.end
  constraint symmetric L86.start L85 L187.end
  constraint symmetric L86.end L85 L188.end
  constraint symmetric L87.start L85 L189.end
  constraint symmetric L87.end L85 L191.end
  constraint symmetric L88.start L85 L190.end
  constraint symmetric L88.end L85 L192.end
  constraint symmetric L89.start L85 L193.end
  constraint vertical L186
  constraint horizontal L182
  constraint vertical L187
  constraint vertical L188
  constraint vertical L189
  constraint vertical L190
  constraint vertical L192
  constraint vertical L193
  constraint collinear L182 L183
  constraint collinear L183 L184
  constraint collinear L184 L185
  constraint vertical L168
  constraint vertical L167
  constraint horizontal L231
  constraint horizontal L234
  constraint coincident L195.end L231
  constraint perpendicular L195 L231
  constraint coincident L138.start L140.end
  constraint horizontal L78
  constraint horizontal L79
  constraint vertical L100
  constraint horizontal L80
  constraint horizontal L81
  constraint horizontal L82
  constraint horizontal L83
  constraint perpendicular L78 L198
  constraint collinear L196 L198
  constraint collinear L197 L198
  constraint collinear L198 L199
  constraint perpendicular L178 L201
  constraint coincident L172.start L201
  constraint collinear L201 L202
  constraint equal L172 L178
  constraint horizontal L70
  constraint horizontal L71
  constraint horizontal L72
  constraint horizontal L73
  constraint horizontal L74
  constraint horizontal L76
  constraint horizontal L133
  constraint horizontal L132
  constraint horizontal L75
  constraint horizontal L131
  constraint horizontal L130
  constraint horizontal L129
  constraint horizontal L128
  constraint horizontal L127
  constraint collinear L109 L127
  constraint collinear L110 L128
  constraint collinear L71 L110
  constraint collinear L111 L129
  constraint collinear L112 L130
  constraint collinear L113 L131
  constraint collinear L114 L132
  constraint collinear L115 L133
  constraint collinear L116 L134
  constraint horizontal L356
  constraint vertical L347
  constraint horizontal L340
  constraint vertical L332
  constraint horizontal L203
  constraint vertical L204
  constraint horizontal L205
  constraint vertical L206
  constraint coincident P8 L207.start
  constraint vertical L373
  constraint horizontal L207
  constraint horizontal L208
  constraint vertical L379
  constraint horizontal L166
  constraint coincident L103.end L166.end
  constraint horizontal L165
  constraint collinear L70 L127
  constraint coincident L90.start L91.start
  constraint perpendicular L77 L218
  constraint collinear L218 L219
  constraint collinear L219 L220
  constraint collinear L220 L221
  constraint vertical L222
  constraint vertical L224
  constraint horizontal L223
  constraint vertical L227
  constraint vertical L225
  constraint vertical L226
  constraint coincident L222.end L517.start
  constraint horizontal L228
  constraint vertical L229
  constraint equal L223 L230
  constraint coincident L136.end L234
  constraint collinear L90 L229
  constraint collinear L168 L224
  constraint collinear L136 L222
  constraint collinear L231 L232
  constraint collinear L233 L234
  constraint vertical L239
  constraint horizontal L236
  constraint coincident L235.start L513.end
  constraint coincident L241.start L513.start
  constraint vertical L240
  constraint perpendicular L236 L242
  constraint vertical L235
  constraint equal L227 L240
  constraint horizontal L243
  constraint vertical L238
  constraint vertical L241
  constraint coincident L138.end L231.end
  constraint horizontal L361
  constraint vertical L244
  constraint horizontal L245
  constraint collinear L103 L244
  constraint horizontal L359
  constraint horizontal L368
  constraint vertical L246
  constraint coincident L229 L368.start
  constraint horizontal L267
  constraint vertical L255
  constraint horizontal L274
  constraint vertical L256
  constraint perpendicular L243 L257
  constraint collinear L267 L269
  constraint collinear L268 L269
  constraint collinear L269 L270
  constraint collinear L271 L274
  constraint collinear L272 L274
  constraint collinear L273 L274
  constraint collinear L274 L275
  constraint vertical L314
  constraint vertical L344
  constraint vertical L320
  constraint vertical L330
  constraint horizontal L335
  constraint horizontal L310
  constraint horizontal L358
  constraint horizontal L316
  constraint collinear L308 L310
  constraint collinear L309 L310
  constraint collinear L310 L311
  constraint collinear L312 L314
  constraint collinear L313 L314
  constraint collinear L314 L315
  constraint collinear L316 L317
  constraint collinear L317 L318
  constraint collinear L318 L319
  constraint collinear L320 L321
  constraint collinear L321 L322
  constraint collinear L322 L323
  constraint collinear L326 L330
  constraint collinear L324 L332
  constraint collinear L324 L325
  constraint collinear L326 L327
  constraint collinear L328 L330
  constraint collinear L329 L332
  constraint collinear L330 L331
  constraint collinear L332 L333
  constraint collinear L334 L340
  constraint collinear L335 L336
  constraint collinear L336 L339
  constraint collinear L337 L340
  constraint collinear L338 L340
  constraint collinear L339 L342
  constraint collinear L340 L341
  constraint collinear L342 L343
  constraint collinear L344 L350
  constraint collinear L345 L347
  constraint collinear L346 L350
  constraint collinear L347 L348
  constraint collinear L348 L352
  constraint collinear L349 L350
  constraint collinear L350 L351
  constraint collinear L352 L353
  constraint collinear L354 L356
  constraint collinear L355 L356
  constraint collinear L356 L357
  constraint collinear L358 L439
  constraint collinear L359 L362
  constraint collinear L360 L361
  constraint collinear L361 L363
  constraint collinear L362 L365
  constraint collinear L363 L364
  constraint collinear L365 L366
  constraint collinear L367 L368
  constraint collinear L368 L369
  constraint collinear L369 L370
  constraint collinear L370 L371
  constraint collinear L372 L379
  constraint collinear L373 L374
  constraint collinear L382 L388
  constraint collinear L374 L377
  constraint collinear L375 L379
  constraint collinear L376 L379
  constraint collinear L377 L378
  constraint collinear L379 L380
  constraint collinear L381 L386
  constraint collinear L382 L383
  constraint collinear L384 L386
  constraint collinear L385 L386
  constraint collinear L386 L387
  constraint collinear L388 L389
  constraint coincident P10 P9
  constraint collinear L390 L402
  constraint collinear L398 L402
  constraint collinear L397 L398
  constraint horizontal L393
  constraint horizontal L392
  constraint vertical L397
  constraint horizontal L395
  constraint horizontal L394
  constraint horizontal L396
  constraint horizontal L399
  constraint horizontal L409
  constraint horizontal L404
  constraint horizontal L391
  constraint horizontal L403
  constraint horizontal L401
  constraint collinear L394 L395
  constraint collinear L396 L399
  constraint collinear L405 L406
  constraint collinear L404 L409
  constraint collinear L403 L407
  constraint collinear L391 L401
  constraint collinear L392 L393
  constraint horizontal L400
  constraint horizontal L411
  constraint vertical L421
  constraint horizontal L412
  constraint vertical L431
  constraint coincident L396.start L421
  constraint coincident L405.start L421
  constraint coincident L409.start L421
  constraint coincident L403.start L421
  constraint coincident L401.start L421
  constraint coincident L410.end L421
  constraint collinear L421 L422
  constraint collinear L422 L423
  constraint collinear L423 L424
  constraint collinear L431 L432
  constraint collinear L432 L433
  constraint collinear L433 L434
  constraint collinear L434 L435
  constraint collinear L78 L413
  constraint collinear L393 L413
  constraint collinear L394 L414
  constraint collinear L396 L415
  constraint collinear L405 L416
  constraint collinear L409 L417
  constraint collinear L403 L418
  constraint collinear L410 L420
  constraint collinear L401 L419
  constraint collinear L408 L420
  constraint collinear L79 L414
  constraint collinear L80 L415
  constraint horizontal L438
  constraint collinear L416 L438
  constraint collinear L81 L417
  constraint collinear L82 L418
  constraint collinear L83 L419
  constraint collinear L84 L420
  constraint collinear L439 L440
  constraint collinear L440 L441
  constraint collinear L441 L442
  constraint coincident L435.end L443.start
  constraint collinear L165 L411
  constraint perpendicular L177 L465
  constraint coincident L458.start L463
  constraint coincident L452.end L465
  constraint perpendicular L458 L465
  constraint perpendicular L453 L463
  constraint coincident L450.end L458
  constraint coincident L451.end L458
  constraint coincident L447.end L458
  constraint coincident L445.end L458
  constraint coincident L444.start L453
  constraint coincident L445.start L453
  constraint coincident L446.start L453
  constraint coincident L447.start L453
  constraint coincident L448.start L453
  constraint coincident L449.start L453
  constraint coincident L451.start L453
  constraint collinear L452 L458
  constraint collinear L453 L455
  constraint collinear L454 L458
  constraint collinear L455 L457
  constraint collinear L456 L458
  constraint collinear L457 L460
  constraint collinear L458 L459
  constraint collinear L460 L461
  constraint coincident L462.end L465
  constraint collinear L463 L464
  constraint collinear L465 L466
  constraint coincident L461 L463.end
  constraint coincident L458 L464.start
  constraint collinear L467 L468
  constraint vertical L469
  constraint horizontal L470
  constraint vertical L471
  constraint vertical L472
  constraint horizontal L473
  constraint vertical L474
  constraint coincident P11 L478.end
  constraint horizontal L476
  constraint collinear L477 L478
  constraint perpendicular L64 L479
  constraint coincident L480.start L479
  constraint collinear L479 L480
  constraint collinear L70 L78
  constraint collinear L209 L290
  constraint collinear L209 L393
  constraint coincident L230.end L245.end
  constraint collinear L483 L487
  constraint collinear L484 L490
  constraint collinear L485 L490
  constraint collinear L486 L487
  constraint collinear L487 L488
  constraint collinear L489 L490
  constraint collinear L490 L491
  constraint horizontal L481
  constraint collinear L443 L481
  constraint perpendicular L411 L497
  constraint collinear L492 L493
  constraint collinear L493 L494
  constraint collinear L494 L495
  constraint collinear L497 L499
  constraint collinear L496 L497
  constraint collinear L497 L498
  constraint collinear L499 L500
  constraint horizontal L510
  constraint vertical L501
  constraint horizontal L508
  constraint vertical L502
  constraint coincident L507.start L506
  constraint collinear L506 L507
  constraint collinear L510 L511
  constraint collinear L512 L513
  constraint collinear L514 L515
  constraint collinear L515 L516
  constraint perpendicular L222 L520
  constraint collinear L518 L519
  constraint collinear L520 L521
  constraint perpendicular L523 L525
  constraint collinear L525 L526
  constraint horizontal L524
  constraint perpendicular L528 L529
  constraint parallel L529 L530
  measures "d12" distance of L7.start P7
  measures "d13" distance of L7.start L15.start
  measures "d19" distance of L7.start L482.start
  measures "d20" distance of L15.start L4.end
  measures "longnotch_l" distance of L2.end L0.start
  measures "d23" distance of L2.end L1.end
  measures "d52" distance of L7.start L2.end
  measures "d60" distance of L4.end L4.start
  measures "d76" diameter of A0
  measures "d77" horizontal distance of L7.start A0.centre
  measures "d78" vertical distance of L7.start A0.centre
  measures "d113" horizontal distance of L7.start L11.start
  measures "d114" vertical distance of L7.start L11.start
  measures "d115" horizontal distance of L16.end L12.end
  measures "d116" vertical distance of L16.end L12.end
  measures "d183" distance of L15.start L15.end
  measures "d270" horizontal distance of L7.start A3.centre
  measures "d271" vertical distance of L15.start A4.centre
  measures "d272" horizontal distance of L15.start A4.centre
  measures "d274" vertical distance of L7.start A3.centre
  measures "sidenub_l" distance of L19.end L17.start
  measures "d278" distance of L19.end L18.end
  measures "d298" distance of L15.start L20.start
  measures "d299" distance of L16.end L16.start
  measures "d348" distance of L17.start L15.end
  measures "d349" distance of L20.end L21.end
  measures "d371" distance of L7.start L482.start
  measures "d411" distance of L5.start L55.start
  measures "d592" distance of L3 L4
  measures "d593" distance of L5 L6
  measures "d607" horizontal distance of L5.start L105.end
  measures "d608" vertical distance of L5.start L105.end
  measures "d677" distance of L85 L104
  measures "d678" distance of L51 L107
  measures "d680" distance of L69 L118
  measures "d681" distance of L63 L66
  measures "d684" distance of L15 L68
  measures "d692" distance of L135.start L135.end
  measures "d693" distance of L135.start L137.start
  measures "d699" distance of L135.start L141.start
  measures "d702" horizontal distance of L141.end L142.start
  measures "d703" vertical distance of L141.end L142.start
  measures "d704" distance of L135.start L135.end
  measures "d705" distance of L147.start L148.start
  measures "d706" distance of L146.end L148.start
  measures "d707" distance of L139.end L151.start
  measures "d710" distance of L139.end L138.start
  measures "d711" distance of L157.start L156.end
  measures "d712" horizontal distance of L155.start L155.end
  measures "d713" vertical distance of L155.start L155.end
  measures "d714" distance of L156.start L156.end
  measures "d715" horizontal distance of L151.end L153.end
  measures "d716" vertical distance of L151.end L153.end
  measures "d718" distance of L145 L153
  measures "d719" distance of L161.end L162.end
  measures "d742" distance of L164.start L168.end
  measures "d743" distance of L167.start L165.start
  measures "d816" distance of L325.end L346.end
  measures "d817" distance of L325.end L330.start
  measures "d820" distance of L206 L332
  measures "d821" distance of L203 L356
  measures "d826" distance of P8 L207.end
  measures "d833" diameter of A15
  measures "d840" horizontal distance of L77.end L77.start
  measures "d841" distance of L224.start L223.end
  measures "d843" distance of L222.end L223